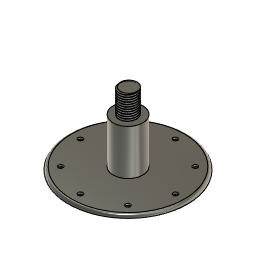
Bottom Panel Mount v6 (Autodesk Fusion 360 design; units mm, degrees)
Autodesk Fusion 360 part; units mm, degrees
sketch "Sketch1" plane through (0, 0, 0) normal (0, 0, 1) x (1, 0, 0)
  circle A0 centre (0, 0) radius 100
  circle A1 centre (80, 0) radius 1.5
  circle A2 centre (0, 0) radius 80
  circle A3 centre (0, 0) radius 80
  circle A4 centre (56.5685, 56.5685) radius 1.5
  circle A5 centre (0, 0) radius 80
  circle A6 centre (0, 80) radius 1.5
  circle A7 centre (0, 0) radius 80
  circle A8 centre (-56.5685, 56.5685) radius 1.5
  circle A9 centre (0, 0) radius 80
  circle A10 centre (-80, 0) radius 1.5
  circle A11 centre (0, 0) radius 80
  circle A12 centre (-56.5685, -56.5685) radius 1.5
  circle A13 centre (0, 0) radius 80
  circle A14 centre (0, -80) radius 1.5
  circle A15 centre (0, 0) radius 80
  circle A16 centre (56.5685, -56.5685) radius 1.5
  dimension "d1" = 200
  dimension "d2" = 3
  dimension "d4" = 360
  dimension "d21" = 160
  constraint coincident A0.centre A2.centre
  constraint concentric A0 A2
  constraint coincident A1.centre A2
  measures "d1" diameter of A0
  measures "d2" diameter of A1
  measures "d21" diameter of A5
extrude "Extrude1" add sketch "Sketch1" along normal blind 5 contours A0 | A1 A2 A3 A4 A5 A6 A7 A8 A9 A10 A11 A12 A13 A14 A15 A16
sketch "Sketch2" plane through (0, 0, 5) normal (0, 0, 1) x (-1, 0, 0)
  circle A0 centre (-80, 0) radius 1.5
  circle A1 centre (56.5685, -56.5685) radius 1.5
  circle A2 centre (-56.5685, -56.5685) radius 1.5
  circle A3 centre (0, -80) radius 1.5
  circle A4 centre (-56.5685, 56.5685) radius 1.5
  circle A5 centre (80, 0) radius 1.5
  circle A6 centre (0, 80) radius 1.5
  circle A7 centre (56.5685, 56.5685) radius 1.5
  circle A8 centre (0, 0) radius 100
  circle A9 centre (-80, 0) radius 4
  circle A10 centre (-56.5685, -56.5685) radius 1.5
  circle A11 centre (-56.5685, -56.5685) radius 4
  circle A12 centre (0, -80) radius 1.5
  circle A13 centre (0, -80) radius 4
  circle A14 centre (56.5685, -56.5685) radius 1.5
  circle A15 centre (56.5685, -56.5685) radius 4
  circle A16 centre (80, 0) radius 1.5
  circle A17 centre (80, 0) radius 4
  circle A18 centre (56.5685, 56.5685) radius 1.5
  circle A19 centre (56.5685, 56.5685) radius 4
  circle A20 centre (0, 80) radius 1.5
  circle A21 centre (0, 80) radius 4
  circle A22 centre (-56.5685, 56.5685) radius 1.5
  circle A23 centre (-56.5685, 56.5685) radius 4
  dimension "d7" = 8
  dimension "d9" = 360
  constraint concentric A0 A9
  measures "d7" diameter of A9
extrude "Extrude2" cut sketch "Sketch2" against normal blind 3 contours A9 | A11 | A13 | A15 | A17 | A19 | A21 | A23
fillet "Fillet1" radius 5 1 edges at (-93.2327, -36.1615, 5)
sketch "Sketch3" plane through (0, 0, 5) normal (0, 0, 1) x (-1, 0, 0)
  circle A0 centre (56.5685, -56.5685) radius 4
  circle A1 centre (-56.5685, 56.5685) radius 4
  circle A2 centre (80, 0) radius 4
  circle A3 centre (-80, 0) radius 4
  circle A4 centre (0, -80) radius 4
  circle A5 centre (0, 80) radius 4
  circle A6 centre (56.5685, 56.5685) radius 4
  circle A7 centre (-56.5685, -56.5685) radius 4
  circle A8 centre (0, 0) radius 95
  circle A9 centre (0, 0) radius 25
  dimension "d13" = 50
  constraint coincident A8.centre A9.centre
  measures "d13" diameter of A9
extrude "Extrude3" add sketch "Sketch3" along normal blind 76 contours A9
sketch "Sketch4" plane through (0, 0, 81) normal (0, 0, 1) x (-1, 0, 0)
  circle A0 centre (0, 0) radius 25
  circle A1 centre (0, 0) radius 15
  dimension "d17" = 30
  constraint concentric A0 A1
  measures "d17" diameter of A1
extrude "Extrude4" add sketch "Sketch4" along normal blind 40 contours A1
thread "Thread2" "ISO Metric profile 30.0 M30x3.5 6g" major diameter 29.7345 minor diameter 25.732 pitch 3.5 angle 60 modelled right hand crest width 0.4992 on face at (-14.9814, 0.7477, 107.6667) crest through (-14.8673, 0, 80.125)
